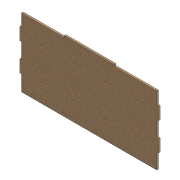
# Autodesk Inventor part: Techo Carcasa
Saved by Autodesk Inventor 2020 (Build 240168000, 168)
## iProperties
Created: 2020-06-04
Part Number: Techo Carcasa
Material: MDF Medium Density Fiberboard
Document SubType Name: Modeling
Designer: Dante
Density: 0.8 g/cm^3
Appearance: Cartón - Ondulado
Mass: 664.312 g
Surface Area: 3112.66 cm^2
Volume: 830.39 cm^3
Author: Dante
Autodesk Inventor part; units mm, degrees
ref_plane "YZ Plane" through (0, 0, 0) normal (1, 0, 0) x (0, 1, 0)
ref_plane "XZ Plane" through (0, 0, 0) normal (0, 1, 0) x (-1, 0, 0)
ref_plane "XY Plane" through (0, 0, 0) normal (0, 0, 1) x (1, 0, 0)
sketch "Sketch1" plane through (0, 0, 0) normal (0, 0, 1) x (1, 0, 0)
  line L0 (456.5044, 429.8855) -> (462.0044, 429.8855)
  line L1 (462.0044, 429.8855) -> (462.0044, 389.8855)
  line L2 (462.0044, 389.8855) -> (456.5044, 389.8855)
  line L3 (456.5044, 389.8855) -> (456.5044, 339.8855)
  line L4 (456.5044, 339.8855) -> (462.0044, 339.8855)
  line L5 (462.0044, 339.8855) -> (462.0044, 339.8855)
  line L6 (22.5044, 429.8855) -> (17.0044, 429.8855)
  line L7 (17.0044, 429.8855) -> (17.0044, 389.8855)
  line L8 (17.0044, 389.8855) -> (22.5044, 389.8855)
  line L9 (22.5044, 389.8855) -> (22.5044, 339.8855)
  line L10 (22.5044, 339.8855) -> (17.0044, 339.8855)
  line L11 (17.0044, 339.8855) -> (17.0044, 339.8855)
  line L12 (17.0044, 339.8855) -> (462.0044, 339.8855)
  line L13 (22.5044, 559.8855) -> (159.5044, 559.8855)
  line L14 (159.5044, 559.8855) -> (159.5044, 565.3855)
  line L15 (456.5044, 559.8855) -> (319.5044, 559.8855)
  line L16 (319.5044, 559.8855) -> (319.5044, 565.3855)
  line L17 (319.5044, 565.3855) -> (159.5044, 565.3855)
  circle A0 centre (174.5044, 552.1705) radius 2
  circle A1 centre (304.5044, 552.1705) radius 2
  line L18 (22.5044, 429.8855) -> (22.5044, 479.8855)
  line L19 (22.5044, 479.8855) -> (17.0044, 479.8855)
  line L20 (17.0044, 479.8855) -> (17.0044, 519.8855)
  line L21 (17.0044, 519.8855) -> (22.5044, 519.8855)
  line L22 (22.5044, 559.8855) -> (22.5044, 519.8855)
  line L23 (22.5044, 479.8855) -> (22.5044, 429.8855)
  line L24 (456.5044, 479.8855) -> (462.0044, 479.8855)
  line L25 (462.0044, 479.8855) -> (462.0044, 519.8855)
  line L26 (462.0044, 519.8855) -> (456.5044, 519.8855)
  line L27 (456.5044, 559.8855) -> (456.5044, 519.8855)
  line L28 (456.5044, 479.8855) -> (456.5044, 429.8855)
  circle A2 centre (105.5044, 349.8855) radius 2
  circle A3 centre (151.0044, 349.8855) radius 2
  circle A4 centre (128.2544, 349.8855) radius 2
  circle A5 centre (328.0044, 349.8855) radius 2
  circle A6 centre (350.7544, 349.8855) radius 2
  circle A7 centre (373.5044, 349.8855) radius 2
  circle A8 centre (31.0044, 504.8855) radius 2
  circle A9 centre (31.0044, 354.8855) radius 2
  circle A10 centre (448.0044, 504.8855) radius 2
  circle A11 centre (448.0044, 354.8855) radius 2
  dimension "d105" = 50
  dimension "d148" = 445
  dimension "d196" = 137
  dimension "d197" = 137
  dimension "d199" = 4
  dimension "d200" = 4
  dimension "d203" = 7.715
  dimension "d204" = 7.715
  dimension "d207" = 5.5
  dimension "d209" = 5.5
  dimension "d211" = 5.5
  dimension "d214" = 4
  dimension "d215" = 4
  dimension "d216" = 4
  dimension "d217" = 4
  dimension "d218" = 4
  dimension "d219" = 4
  dimension "d221" = 22.75
  dimension "d222" = 22.75
  dimension "d224" = 22.75
  dimension "d225" = 22.75
  dimension "d226" = 4
  dimension "d227" = 4
  dimension "d234" = 90
  dimension "d235" = 90
  dimension "d236" = 90
  dimension "d238" = 55
  dimension "d244" = 160
  dimension "d245" = 5.5
  dimension "d246" = 5.5
  dimension "d247" = 5.5
  dimension "d248" = 5.5
  dimension "d249" = 5.5
  dimension "d250" = 5.5
  dimension "d251" = 8.5
  dimension "d252" = 8.5
  dimension "d253" = 150
  dimension "d254" = 152
  dimension "d255" = 152
  dimension "d256" = 55
  dimension "d257" = 8.5
  dimension "d258" = 4
  dimension "d259" = 8.5
  dimension "d260" = 150
  dimension "d261" = 10
  dimension "d262" = 10
  dimension "d263" = 10
  dimension "d264" = 10
  dimension "d265" = 10
  dimension "d266" = 10
  dimension "d269" = 40
  dimension "d270" = 40
  dimension "d271" = 40
  dimension "d272" = 50
  dimension "d273" = 40
  dimension "d274" = 40
  dimension "d275" = 50
  dimension "d276" = 40
  dimension "d277" = 50
  dimension "d280" = 0
  dimension "d281" = 0
  dimension "d282" = 0
  dimension "d283" = 90
  dimension "d284" = 90
  constraints: 58 end point, 15 perpendicular, 12 centre point, 5 vertical, 3 point on line, 2 parallel
  measures "d105" distance of L2.end L3.end
  measures "d148" distance of L11.end L5.end
  measures "d196" distance of L13.start L13.end
  measures "d197" distance of L15.start L15.end
  measures "d199" diameter of A0
  measures "d200" diameter of A1
  measures "d203" distance from line of L13 A0.centre
  measures "d204" distance from line of L15 A1.centre
  measures "d207" distance between parallel lines of L15 L17
  measures "d209" distance of L18.end L19.end
  measures "d211" distance of L24.start L24.end
  measures "d214" diameter of A2
  measures "d215" diameter of A3
  measures "d216" diameter of A4
  measures "d217" diameter of A5
  measures "d218" diameter of A6
  measures "d219" diameter of A7
  measures "d221" distance of A6.centre A7.centre
  measures "d222" distance of A5.centre A6.centre
  measures "d224" distance of A2.centre A4.centre
  measures "d225" distance of A3.centre A4.centre
  measures "d226" diameter of A8
  measures "d227" diameter of A9
  measures "d234" angle of L22 L13
  measures "d235" angle of L12 L11
  measures "d236" angle of L27 L15
  measures "d238" distance from line of L13 A8.centre
  measures "d244" distance of L16.end L14.end
  measures "d245" distance of L6.start L6.end
  measures "d246" distance of L9.end L10.end
  measures "d247" distance of L7.end L8.end
  measures "d248" distance of L20.end L21.end
  measures "d249" distance of L0.start L0.end
  measures "d250" distance of L3.end L4.end
  measures "d251" distance from line of L18 A8.centre
  measures "d252" distance from line of L9 A9.centre
  measures "d253" distance of A9.centre A8.centre
  measures "d254" distance from line of L22 A0.centre
  measures "d255" distance from line of L27 A1.centre
  measures "d256" distance from line of L15 A10.centre
  measures "d257" distance from line of L27 A10.centre
  measures "d258" diameter of A11
  measures "d259" distance from line of L3 A11.centre
  measures "d260" distance of A10.centre A11.centre
  measures "d261" distance from line of L12 A7.centre
  measures "d262" distance from line of L12 A6.centre
  measures "d263" distance from line of L12 A5.centre
  measures "d264" distance from line of L12 A3.centre
  measures "d265" distance from line of L12 A4.centre
  measures "d266" distance from line of L12 A2.centre
  measures "d269" distance of L13.start L21.end
  measures "d270" distance of L15.start L26.end
  measures "d271" distance of L24.end L25.end
  measures "d272" distance of L24.start L0.start
  measures "d273" distance of L0.end L1.end
  measures "d274" distance of L19.end L20.end
  measures "d275" distance of L18.end L6.start
  measures "d276" distance of L6.end L7.end
  measures "d277" distance of L8.end L9.end
  measures "d280" distance of L4.end L5.end
  measures "d281" distance of L10.end L11.end
  measures "d282" distance between parallel lines of L12 L10
  measures "d283" angle of L12 L3
  measures "d284" angle of L8 L7
extrude "Extrusion1" add sketch "Sketch1" along normal blind 5.5
body "Solid1"
